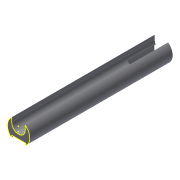
# Autodesk Inventor part: Slotted center beam_xw
Saved by Autodesk Inventor 2016 (Build 200138000, 138)
## iProperties
Created: 2013-10-22
Part Number: Slotted center beam_xw
Document SubType Name: Modeling
Designer: 121767
Density: 1 g/cm^3
Material: Generic
Appearance: Default
Author: 121767
Autodesk Inventor part; units mm, degrees
ref_plane "YZ Plane" through (0, 0, 0) normal (1, 0, 0) x (0, 1, 0)
ref_plane "XZ Plane" through (0, 0, 0) normal (0, 1, 0) x (-1, 0, 0)
ref_plane "XY Plane" through (0, 0, 0) normal (0, 0, 1) x (1, 0, 0)
sketch "Sketch1" plane through (0, 0, 0) normal (0, 0, 1) x (1, 0, 0)
  line L0 (-2.5114, -3.0648) -> (-2.5114, -2.286)
  line L1 (-2.5114, -2.286) -> (2.5686, -2.286)
  line L2 (2.5686, -2.286) -> (2.5686, -3.0171)
  line L3 (0.0286, -2.286) -> (0.0286, -6.1579) construction
  arc A0 (-2.4226, 1.5748) -> (2.3526, 1.5748) centre (-0.035, 1.5748) ccw
  line L4 (-0.035, 1.5748) -> (2.3526, 1.5748) construction
  line L5 (-0.035, 1.5748) -> (-2.4226, 1.5748) construction
  line L6 (-2.4226, 1.5748) -> (-2.4226, 3.1356)
  line L7 (2.3526, 1.5748) -> (2.3526, 3.1884)
  line L8 (-1.9936, 0) -> (0, 0)
  arc A1 (2.5686, -3.0171) -> (2.3526, 3.1884) centre (0, 0) ccw
  arc A2 (-2.4226, 3.1356) -> (-2.5114, -3.0648) centre (0, 0) ccw
  point P0 (-2.54, -2.286)
  point P1 (2.54, -2.286)
  dimension "d14" = 5.08
  dimension "d22" = 2.3876
  dimension "d31" = 2.286
  dimension "d32" = 1.5748
  dimension "d36" = 3.9624
  dimension "d37" = 3.9624
  constraints: 18 end point, 6 point on circle, 3 centre point, 3 parallel, 2 point on line, 2 tangent, 1 coincident, 1 horizontal, 1 midpoint, 1 vertical, 1 other
  measures "d14" distance between parallel lines of L2 L0
  measures "d22" radius of A0
  measures "d31" distance between parallel lines of L8 L1
  measures "d32" distance from line of point (0, 0) L4
  measures "d36" radius of A1
  measures "d37" radius of A2
extrude "Extrusion4" add sketch "Sketch1" along normal blind 50.8
sketch "Sketch2" plane through (0, 0, 0) normal (0, 0, -1) x (-1, 0, 0)
  line L0 (2.5114, -3.0648) -> (2.5114, -2.286) projected
  line L1 (-2.5686, -2.286) -> (-2.5686, -3.0171) projected
  line L2 (2.5114, -3.0648) -> (2.5114, -2.286) projected
  line L3 (2.5114, -2.286) -> (2.5114, 0.3388)
  line L4 (2.5114, 0.3388) -> (-2.5686, 0.3388)
  line L5 (-2.5686, -2.286) -> (-2.5686, -3.0171) projected
  line L6 (-2.5686, 0.3388) -> (-2.5686, -2.286)
  point P0 (0, 0)
  dimension "d24" = 3.4036
  constraints: 6 end point, 2 collinear, 2 perpendicular, 1 vertical
  measures "d24" distance of L3.end L0.start
extrude "Extrusion5" cut sketch "Sketch2" against normal blind 10 fills toward (2.4614, -0.9736) open curves L3 L4 L6
sketch "Sketch4" plane through (0, 0, 50.8) normal (0, 0, 1) x (1, 0, 0)
  line L0 (-2.5114, -3.0648) -> (-2.5114, -2.286) projected
  line L1 (-2.5114, -2.286) -> (2.5686, -2.286) projected
  line L2 (2.5686, -2.286) -> (2.5686, -3.0171) projected
  arc A0 (2.5686, -3.0171) -> (2.3526, 3.1884) centre (0, 0) ccw projected
  line L3 (2.3526, 3.1884) -> (2.3526, 1.5748) projected
  arc A1 (-2.4226, 1.5748) -> (2.3526, 1.5748) centre (-0.035, 1.5748) ccw projected
  line L4 (-2.4226, 1.5748) -> (-2.4226, 3.1356) projected
  arc A2 (-2.4226, 3.1356) -> (-2.5114, -3.0648) centre (0, 0) ccw projected
body "Solid3"
